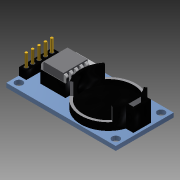
# Autodesk Inventor part: REAL_TIME_SHEELD
Saved by Autodesk Inventor 2014 SP1 (Build 180222100, 222)
## iProperties
Created: 2015-12-16
Part Number: REAL_TIME_SHEELD
Material: Типовые
Document SubType Name: Modeling
Designer: Oleg
Density: 1 g/cm^3
Appearance: По умолчанию
Author: Oleg
Autodesk Inventor part; units mm, degrees
note: some values were not read from the file. Chosen so that the rebuilt part matches the saved one: sketch regions of "Выдавливание14".
ref_plane "YZ Plane" through (0, 0, 0) normal (1, 0, 0) x (0, 1, 0)
ref_plane "XZ Plane" through (0, 0, 0) normal (0, 1, 0) x (-1, 0, 0)
ref_plane "XY Plane" through (0, 0, 0) normal (0, 0, 1) x (1, 0, 0)
sketch "Эскиз1" plane through (0, 0, 0) normal (0, 0, 1) x (1, 0, 0)
  line L0 (-21.75, 11.5) -> (21.75, 11.5)
  line L1 (21.75, 11.5) -> (21.75, -11.5)
  line L2 (21.75, -11.5) -> (-21.75, -11.5)
  line L3 (-21.75, -11.5) -> (-21.75, 11.5)
  line L4 (-21.75, 11.5) -> (21.75, -11.5) construction
  line L5 (-21.75, -11.5) -> (21.75, 11.5) construction
  circle A0 centre (-19.25, 9) radius 1.5
  circle A1 centre (19.25, 9) radius 1.5
  circle A2 centre (-19.25, -9) radius 1.5
  circle A3 centre (19.25, -9) radius 1.5
  point P0 (0, 0)
  point P1 (0, 0)
  dimension "d0" = 43.5
  dimension "d1" = 23
  dimension "d4" = 38.5
  dimension "d5" = 3
  dimension "d6" = 3
  dimension "d7" = 38.5
  dimension "d8" = 18
  dimension "d9" = 18
  dimension "d10" = 2.5
  dimension "d11" = 2.5
  dimension "d12" = 2.5
  dimension "d13" = 2.5
  constraints: 12 end point, 4 centre point, 2 equal radius, 2 parallel, 1 coincident, 1 horizontal, 1 midpoint, 1 perpendicular
  measures "d0" distance of L0.start L0.end
  measures "d1" distance of L0.end L1.end
  measures "d4" distance of A1.centre A0.centre
  measures "d5" diameter of A1
  measures "d6" diameter of A0
  measures "d7" distance of A3.centre A2.centre
  measures "d8" distance of A0.centre A2.centre
  measures "d9" distance of A3.centre A1.centre
  measures "d10" distance from line of L1 A1.centre
  measures "d11" distance from line of L0 A1.centre
  measures "d12" distance from line of L0 A0.centre
  measures "d13" distance from line of L3 A2.centre
extrude "Выдавливание2" add sketch "Эскиз1" along normal blind 1.7
sketch "Эскиз2" plane through (0, 0, 1.7) normal (0, 0, 1) x (1, 0, 0)
  line L0 (21.75, 11.5) -> (-21.75, 11.5)
  line L1 (-21.75, 11.5) -> (-21.75, -11.5)
  line L2 (-21.75, -11.5) -> (21.75, -11.5)
  line L3 (21.75, -11.5) -> (21.75, 11.5)
  arc A0 (17.75, 3.5) -> (17.75, -3.5) centre (7.321673, 0) ccw
  line L4 (17.75, 3.5) -> (20.75, 3.5)
  line L5 (20.75, 3.5) -> (20.75, -3.5)
  line L6 (20.75, -3.5) -> (17.75, -3.5)
  line L7 (-14.75, 5) -> (-4.75, 5)
  line L8 (-4.75, 5) -> (-4.75, -5)
  line L9 (-4.75, -5) -> (-14.75, -5)
  line L10 (-14.75, -5) -> (-14.75, 5)
  point P0 (0, 0)
  dimension "d16" = 22
  dimension "d18" = 8
  dimension "d19" = 8
  dimension "d20" = 1
  dimension "d21" = 10
  dimension "d22" = 10
  dimension "d23" = 7
  dimension "d24" = 3
  dimension "d25" = 6.5
  constraints: 14 end point, 4 parallel, 2 horizontal, 2 perpendicular, 2 point on circle, 1 centre point
  measures "d16" diameter of A0
  measures "d18" distance between parallel lines of L0 L4
  measures "d19" distance between parallel lines of L2 L6
  measures "d20" distance between parallel lines of L3 L5
  measures "d21" distance of L7.start L7.end
  measures "d22" distance of L9.end L7.start
  measures "d23" distance between parallel lines of L1 L10
  measures "d24" distance of L5.end L6.end
  measures "d25" distance between parallel lines of L0 L7
extrude "Выдавливание3" add sketch "Эскиз2" along normal blind 8 contours L4 L5 L6 A0 | L7 L8 L9 L10
sketch "Эскиз3" plane through (0, 0, 9.7) normal (0, 0, 1) x (1, 0, 0)
  arc A0 (17.75, 3.5) -> (17.75, -3.5) centre (7.321673, 0) ccw
  line L0 (17.75, -3.5) -> (20.75, -3.5)
  line L1 (20.75, -3.5) -> (20.75, 3.5)
  line L2 (20.75, 3.5) -> (17.75, 3.5)
  circle A1 centre (7.321673, 0) radius 10
  line L3 (19.75, 2.5) -> (17.75, 2.5)
  line L4 (17.75, 2.5) -> (17.75, -2.5)
  line L5 (17.75, -2.5) -> (19.75, -2.5)
  line L6 (19.75, -2.5) -> (19.75, 2.5)
  point P0 (0, 0)
  dimension "d28" = 20
  dimension "d29" = 1
  dimension "d30" = 1
  dimension "d31" = 1
  dimension "d32" = 2
  constraints: 8 end point, 2 parallel, 1 centre point, 1 coincident, 1 horizontal, 1 perpendicular
  measures "d28" diameter of A1
  measures "d29" distance between parallel lines of L3 L2
  measures "d30" distance between parallel lines of L0 L5
  measures "d31" distance between parallel lines of L1 L6
  measures "d32" distance between parallel lines of L6 L4
extrude "Выдавливание4" cut sketch "Эскиз3" against normal blind 7 contours A1 | L6 L5 L4 L3
sketch "Эскиз4" plane through (0, 0, 9.7) normal (0, 0, 1) x (1, 0, 0)
  circle A0 centre (7.321673, 0) radius 10
  arc A1 (17.75, 3.5) -> (17.75, -3.5) centre (7.321673, 0) ccw
  line L0 (-1.209908, 6.943495) -> (-0.392903, 6.362807)
  line L1 (15.036249, 6.362807) -> (15.853255, 6.943495)
  line L2 (15.036249, -6.362807) -> (15.853255, -6.943495)
  line L3 (-1.651324, -6.362807) -> (-0.83623, -5.783478)
  point P0 (0, 0)
  constraints: 8 end point, 8 point on circle, 2 parallel
extrude "Выдавливание5" cut sketch "Эскиз4" against normal blind 5 contours A0 L0 A1 L1 | L2 A1 L3 A0
sketch "Эскиз5" plane through (0, 0, 9.7) normal (0, 0, 1) x (1, 0, 0)
  line L0 (-4.75, 5) -> (-14.75, 5) projected
  line L1 (-14.75, 5) -> (-14.75, -5) projected
  line L2 (-14.75, -5) -> (-4.75, -5) projected
  line L3 (-4.75, -5) -> (-4.75, 5) projected
  line L4 (-13.75, 4.8) -> (-5.75, 4.8)
  line L5 (-5.75, 4.8) -> (-5.75, -4.8)
  line L6 (-5.75, -4.8) -> (-13.75, -4.8)
  line L7 (-13.75, -4.8) -> (-13.75, 4.8)
  point P0 (0, 0)
  dimension "d37" = 0.2
  dimension "d38" = 0.2
  dimension "d39" = 1
  dimension "d40" = 1
  constraints: 8 end point, 2 parallel, 1 horizontal, 1 perpendicular
  measures "d37" distance between parallel lines of L0 L4
  measures "d38" distance between parallel lines of L2 L6
  measures "d39" distance between parallel lines of L7 L1
  measures "d40" distance between parallel lines of L3 L5
extrude "Выдавливание6" cut sketch "Эскиз5" against normal blind 3
sketch "Эскиз6" plane through (0, 0, 1.7) normal (0, 0, 1) x (1, 0, 0)
  line L0 (-14.75, 5) -> (-4.75, 5)
  line L1 (-21.75, 11.5) -> (-21.75, -11.5)
  line L2 (-15.75, 10.5) -> (-7.75, 10.5)
  line L3 (-7.75, 10.5) -> (-7.75, 7.5) construction
  line L4 (-7.75, 7.5) -> (-15.75, 7.5)
  line L5 (-15.75, 7.5) -> (-15.75, 10.5) construction
  arc A0 (-15.75, 10.5) -> (-15.75, 7.5) centre (-15.027774, 9) ccw
  arc A1 (-7.75, 7.5) -> (-7.75, 10.5) centre (-7.75, 9) ccw
  point P0 (0, 0)
  dimension "d43" = 3
  dimension "d44" = 2.5
  dimension "d45" = 6
  dimension "d46" = 8
  constraints: 8 end point, 4 point on circle, 2 centre point, 2 parallel, 2 tangent, 1 horizontal, 1 perpendicular
  measures "d43" distance between parallel lines of L4 L2
  measures "d44" distance between parallel lines of L0 L4
  measures "d45" distance between parallel lines of L1 L5
  measures "d46" distance between parallel lines of L3 L5
extrude "Выдавливание7" add sketch "Эскиз6" along normal blind 3
sketch "Эскиз7" plane through (0, 0, 1.7) normal (0, 0, 1) x (1, 0, 0)
  circle A0 centre (-19.25, -9) radius 1.5 projected
  circle A1 centre (-19.25, 9) radius 1.5 projected
  line L0 (-21.75, 11.5) -> (-21.75, -11.5) projected
  line L1 (21.75, -11.5) -> (21.75, 11.5) projected
  line L2 (-19.25, 9) -> (-19.25, -9) construction
  circle A2 centre (-20.25, 5.08) radius 0.75
  line L3 (-19.25, 6.46) -> (-19.25, -11.54) construction
  circle A3 centre (-20.25, 2.54) radius 0.75
  line L4 (-19.25, 3.92) -> (-19.25, -14.08) construction
  circle A4 centre (-20.25, 0) radius 0.75
  line L5 (-19.25, 1.38) -> (-19.25, -16.62) construction
  circle A5 centre (-20.25, -2.54) radius 0.75
  line L6 (-19.25, -1.16) -> (-19.25, -19.16) construction
  circle A6 centre (-20.25, -5.08) radius 0.75
  point P0 (0, 0)
  dimension "d49" = 1.5
  dimension "d50" = 1.5
  dimension "d53" = 2.54
  dimension "d58" = 3.92
  constraints: 10 end point, 5 centre point, 1 collinear, 1 parallel, 1 vertical, 19 other
  measures "d49" diameter of A2
  measures "d50" distance from line of A2.centre L0
  measures "d53" distance of A2.centre A3.centre
  measures "d58" vertical distance of L2.start A2.centre
extrude "Выдавливание8" cut sketch "Эскиз7" against normal blind 1.7 contours A2 | A3 | A4 | A5 | A6
sketch "Эскиз8" plane through (0, 0, 9.7) normal (0, 0, 1) x (1, 0, 0)
  line L0 (-13.75, 4.8) -> (-13.75, -4.8) projected
  line L1 (-5.75, 4.8) -> (-13.75, 4.8) projected
  line L2 (-13.75, 4.8) -> (-13.75, -4.8) construction
  line L3 (-5.75, 4.8) -> (-13.75, 4.8) construction
  line L4 (-5.75, -4.8) -> (-5.75, 4.8) construction
  line L5 (-13.75, -4.8) -> (-5.75, -4.8) construction
  line L6 (-14.75, 5) -> (-4.75, 5) construction
  line L7 (-14.75, -5) -> (-14.75, 5) construction
  line L8 (-4.75, -5) -> (-14.75, -5) construction
  line L9 (-4.75, 5) -> (-4.75, -5) construction
  line L10 (-13.75, 4.5) -> (-14.75, 4.5)
  line L11 (-14.75, 4.5) -> (-14.75, 3.5)
  line L12 (-14.75, 3.5) -> (-13.75, 3.5)
  line L13 (-13.75, 3.5) -> (-13.75, 4.5)
  line L14 (-13.75, 2.46) -> (-14.75, 2.46)
  line L15 (-14.75, 2.46) -> (-14.75, 1.46)
  line L16 (-14.75, 1.46) -> (-13.75, 1.46)
  line L17 (-13.75, 1.46) -> (-13.75, 2.46)
  line L18 (-13.75, 0.42) -> (-14.75, 0.42)
  line L19 (-14.75, 0.42) -> (-14.75, -0.58)
  line L20 (-14.75, -0.58) -> (-13.75, -0.58)
  line L21 (-13.75, -0.58) -> (-13.75, 0.42)
  line L22 (-13.75, -1.62) -> (-14.75, -1.62)
  line L23 (-14.75, -1.62) -> (-14.75, -2.62)
  line L24 (-14.75, -2.62) -> (-13.75, -2.62)
  line L25 (-13.75, -2.62) -> (-13.75, -1.62)
  line L26 (-13.75, -3.66) -> (-14.75, -3.66)
  line L27 (-14.75, -3.66) -> (-14.75, -4.66)
  line L28 (-14.75, -4.66) -> (-13.75, -4.66)
  line L29 (-13.75, -4.66) -> (-13.75, -3.66)
  line L30 (-4.75, 4.5) -> (-5.75, 4.5)
  line L31 (-5.75, 4.5) -> (-5.75, 3.5)
  line L32 (-5.75, 3.5) -> (-4.75, 3.5)
  line L33 (-4.75, 3.5) -> (-4.75, 4.5)
  line L34 (-4.75, 1.46) -> (-4.75, 2.46)
  line L35 (-5.75, 2.46) -> (-5.75, 1.46)
  line L36 (-5.75, 1.46) -> (-4.75, 1.46)
  line L37 (-4.75, 2.46) -> (-5.75, 2.46)
  line L38 (-4.75, -0.58) -> (-4.75, 0.42)
  line L39 (-5.75, 0.42) -> (-5.75, -0.58)
  line L40 (-5.75, -0.58) -> (-4.75, -0.58)
  line L41 (-4.75, 0.42) -> (-5.75, 0.42)
  line L42 (-4.75, -2.62) -> (-4.75, -1.62)
  line L43 (-5.75, -1.62) -> (-5.75, -2.62)
  line L44 (-5.75, -2.62) -> (-4.75, -2.62)
  line L45 (-4.75, -1.62) -> (-5.75, -1.62)
  line L46 (-4.75, -4.66) -> (-4.75, -3.66)
  line L47 (-5.75, -3.66) -> (-5.75, -4.66)
  line L48 (-5.75, -4.66) -> (-4.75, -4.66)
  line L49 (-4.75, -3.66) -> (-5.75, -3.66)
  point P0 (0, 0)
  point P1 (-4.75, 4.8)
  point P2 (-4.75, -4.8)
  point P3 (-4.75, -4.8)
  point P4 (-4.75, 4.8)
  point P5 (-5.75, 5)
  point P6 (-5.75, -5)
  dimension "d61" = 1
  dimension "d62" = 0.3
  dimension "d65" = 2.04
  dimension "d72" = 9
  constraints: 80 end point, 2 horizontal, 2 parallel, 2 point on line, 1 perpendicular, 1 vertical, 78 other
  measures "d61" distance of L12.end L10.start
  measures "d62" distance between parallel lines of L3 L10
  measures "d65" distance of L10.start L17.end
  measures "d72" distance of L0.start point (-4.75, 4.8)
extrude "Выдавливание9" add sketch "Эскиз8" against normal blind 3
fillet "Сопряжение1" radius 1 4 edges at (-6.25, 9, 4.7) (-11.75, 7.5, 4.7) (-11.75, 10.5, 4.7) (-16.6926, 9, 4.7)
sketch "Эскиз9" plane through (0, 0, 1.7) normal (0, 0, 1) x (1, 0, 0)
  circle A0 centre (-20.25, -2.54) radius 0.75 projected
  circle A1 centre (-20.25, 2.54) radius 0.75 projected
  circle A2 centre (-20.25, 5.08) radius 0.75 projected
  circle A3 centre (-20.25, 0) radius 0.75 projected
  circle A4 centre (-20.25, -5.08) radius 0.75 projected
  line L0 (-21.75, 11.5) -> (-21.75, -11.5) projected
  line L1 (-21.75, 6.58) -> (-18.75, 6.58)
  line L2 (-18.75, 6.58) -> (-18.75, -6.58)
  line L3 (-18.75, -6.58) -> (-21.75, -6.58)
  line L4 (-21.75, -6.58) -> (-21.75, 6.58)
  point P0 (0, 0)
  dimension "d80" = 3
  dimension "d81" = 1.5
  dimension "d82" = 1.5
  constraints: 8 end point, 2 parallel, 1 horizontal, 1 perpendicular, 1 point on line
  measures "d80" distance between parallel lines of L2 L0
  measures "d81" distance from line of L1 A2.centre
  measures "d82" distance from line of L3 A4.centre
extrude "Выдавливание10" add sketch "Эскиз9" along normal blind 3
sketch "Эскиз10" plane through (0, 0, 4.7) normal (0, 0, 1) x (1, 0, 0)
  circle A0 centre (-20.25, -5.08) radius 0.75 projected
  circle A1 centre (-20.25, 0) radius 0.75 projected
  circle A2 centre (-20.25, 5.08) radius 0.75 projected
  circle A3 centre (-20.25, 2.54) radius 0.75 projected
  circle A4 centre (-20.25, -2.54) radius 0.75 projected
  circle A5 centre (-20.25, 5.08) radius 0.5
  circle A6 centre (-20.25, 2.54) radius 0.5
  circle A7 centre (-20.25, 0) radius 0.5
  circle A8 centre (-20.25, -2.54) radius 0.5
  circle A9 centre (-20.25, -5.08) radius 0.5
  point P0 (0, 0)
  dimension "d85" = 1
  constraints: 5 centre point, 5 coincident, 4 equal radius
  measures "d85" diameter of A5
extrude "Выдавливание11" add sketch "Эскиз10" along normal blind 5 contours A5 | A6 | A7 | A8 | A9
sketch "Эскиз11" plane through (0, 0, 0) normal (0, 0, -1) x (-1, 0, 0)
  circle A0 centre (20.25, 5.08) radius 0.5 projected
  circle A1 centre (20.25, 2.54) radius 0.5 projected
  circle A2 centre (20.25, 0) radius 0.5 projected
  circle A3 centre (20.25, -2.54) radius 0.5 projected
  circle A4 centre (20.25, -5.08) radius 0.5 projected
  point P0 (0, 0)
extrude "Выдавливание12" add sketch "Эскиз11" along normal blind 1
sketch "Эскиз12" plane through (7.321673, 0, 2.7) normal (0, 0, 1) x (1, 0, 0)
  circle A0 centre (0, 0) radius 10
  line L0 (9.337266, 3.05809) -> (9.453069, 3.05809)
  line L1 (9.453069, 3.05809) -> (9.453069, -3.261822)
  line L2 (9.453069, -3.261822) -> (9.337266, -3.261822)
  line L3 (9.337266, -3.261822) -> (9.337266, 3.05809)
  point P0 (-7.321673, 0)
  constraints: 8 end point, 2 parallel, 1 horizontal, 1 perpendicular, 2 other
extrude "Выдавливание13" add sketch "Эскиз12" along normal blind 5 contours L2 L3 L0 L1
sketch "Эскиз13" plane through (0, 0, 9.7) normal (0, 0, 1) x (1, 0, 0)
  line L0 (-13.75, 4.8) -> (-13.75, 4.5) projected
  line L1 (-13.75, 4.5) -> (-14.75, 4.5) projected
  line L2 (-14.75, 4.5) -> (-14.75, 3.5) projected
  line L3 (-14.75, 3.5) -> (-13.75, 3.5) projected
  line L4 (-13.75, 3.5) -> (-13.75, 2.46) projected
  line L5 (-13.75, 2.46) -> (-14.75, 2.46) projected
  line L6 (-14.75, 2.46) -> (-14.75, 1.46) projected
  line L7 (-14.75, 1.46) -> (-13.75, 1.46) projected
  line L8 (-13.75, 1.46) -> (-13.75, 0.42) projected
  line L9 (-13.75, 0.42) -> (-14.75, 0.42) projected
  line L10 (-14.75, 0.42) -> (-14.75, -0.58) projected
  line L11 (-14.75, -0.58) -> (-13.75, -0.58) projected
  line L12 (-13.75, -0.58) -> (-13.75, -1.62) projected
  line L13 (-13.75, -1.62) -> (-14.75, -1.62) projected
  line L14 (-14.75, -1.62) -> (-14.75, -2.62) projected
  line L15 (-14.75, -2.62) -> (-13.75, -2.62) projected
  line L16 (-13.75, -2.62) -> (-13.75, -3.66) projected
  line L17 (-13.75, -3.66) -> (-14.75, -3.66) projected
  line L18 (-14.75, -3.66) -> (-14.75, -4.66) projected
  line L19 (-14.75, -4.66) -> (-13.75, -4.66) projected
  line L20 (-13.75, -4.66) -> (-13.75, -4.8) projected
  line L21 (-13.75, -4.8) -> (-5.75, -4.8) projected
  line L22 (-5.75, -4.8) -> (-5.75, -4.66) projected
  line L23 (-5.75, -4.66) -> (-4.75, -4.66) projected
  line L24 (-4.75, -4.66) -> (-4.75, -3.66) projected
  line L25 (-4.75, -3.66) -> (-5.75, -3.66) projected
  line L26 (-5.75, -3.66) -> (-5.75, -2.62) projected
  line L27 (-5.75, -2.62) -> (-4.75, -2.62) projected
  line L28 (-4.75, -2.62) -> (-4.75, -1.62) projected
  line L29 (-4.75, -1.62) -> (-5.75, -1.62) projected
  line L30 (-5.75, -1.62) -> (-5.75, -0.58) projected
  line L31 (-4.75, -0.58) -> (-5.75, -0.58) projected
  line L32 (-4.75, 0.42) -> (-4.75, -0.58) projected
  line L33 (-5.75, 0.42) -> (-4.75, 0.42) projected
  line L34 (-5.75, 0.42) -> (-5.75, 1.46) projected
  line L35 (-4.75, 1.46) -> (-5.75, 1.46) projected
  line L36 (-4.75, 2.46) -> (-4.75, 1.46) projected
  line L37 (-5.75, 2.46) -> (-4.75, 2.46) projected
  line L38 (-5.75, 2.46) -> (-5.75, 3.5) projected
  line L39 (-4.75, 3.5) -> (-5.75, 3.5) projected
  line L40 (-4.75, 4.5) -> (-4.75, 3.5) projected
  line L41 (-5.75, 4.5) -> (-4.75, 4.5) projected
  line L42 (-5.75, 4.5) -> (-5.75, 4.8) projected
  line L43 (-5.75, 4.8) -> (-13.75, 4.8) projected
  line L44 (-5.75, 4.5) -> (-5.75, -4.66)
  line L45 (-13.75, 4.5) -> (-13.75, -4.8)
  point P0 (0, 0)
  constraints: 4 end point, 1 parallel, 1 perpendicular
extrude "Выдавливание14" cut sketch "Эскиз13" against normal blind 0.5 contours L45 L3 L2 L1 | L41 L40 L39 L44 | L45 L7 L6 L5 | L37 L36 L35 L44 | L45 L11 L10 L9 | L33 L32 L31 L44 | L45 L15 L14 L13 | L29 L28 L27 L44 | L45 L19 L18 L17 | L25 L24 L23 L44
fillet "Сопряжение2" radius 1 10 edges at (-14.75, 4, 9.2) (-14.75, 1.96, 9.2) (-14.75, -0.08, 9.2) (-14.75, -2.12, 9.2) (-14.75, -4.16, 9.2) (-4.75, -4.16, 9.2) (-4.75, -2.12, 9.2) (-4.75, -0.08, 9.2) (-4.75, 1.96, 9.2) (-4.75, 4, 9.2)
sketch "Эскиз14" plane through (-21.75, -11.5, 0) normal (-1, 0, 0) x (0, 0, 1)
  line L0 (1.7, 4.92) -> (4.7, 4.92) projected
  line L1 (4.7, 18.08) -> (4.7, 4.92) projected
  line L2 (1.7, 18.08) -> (4.7, 18.08) projected
  line L3 (0, 23) -> (1.7, 23) projected
  line L4 (1.7, 18.08) -> (1.7, 4.92)
  point P0 (0, 11.5)
  constraints: 2 end point, 1 perpendicular
extrude "Выдавливание15" cut sketch "Эскиз14" against normal blind 0.1
